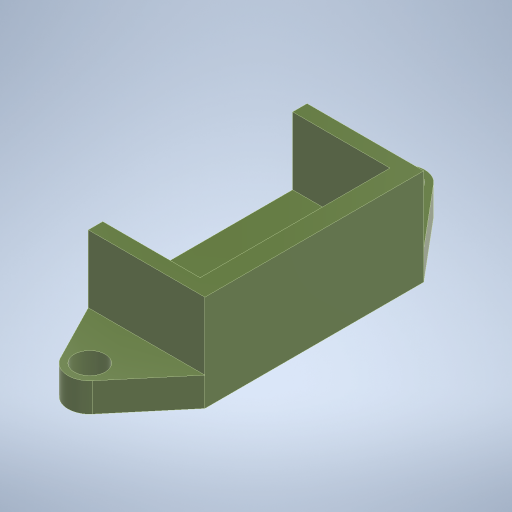
# Autodesk Inventor part: креп_концевика
Saved by Autodesk Inventor 2023.1 (Build 271208000, 208)
## iProperties
Created: 2026-01-30
Part Number: креп_концевика
Material: Типовые
Document SubType Name: Modeling
Designer: DELL
Density: 1 g/cm^3
Appearance: Темно-оливковый
Author: DELL
Autodesk Inventor part; units mm, degrees
ref_plane "YZ Plane" through (0, 0, 0) normal (1, 0, 0) x (0, 1, 0)
ref_plane "XZ Plane" through (0, 0, 0) normal (0, 1, 0) x (-1, 0, 0)
ref_plane "XY Plane" through (0, 0, 0) normal (0, 0, 1) x (1, 0, 0)
sketch "Эскиз1" plane through (0, 0, 0) normal (0, 1, 0) x (-1, 0, 0)
  line L0 (5.05, 9.85) -> (-5.05, 9.85)
  line L1 (-5.05, 9.85) -> (-5.05, -9.85)
  line L2 (-5.05, -9.85) -> (5.05, -9.85)
  line L3 (5.05, -9.85) -> (5.05, 9.85)
  line L4 (5.05, 9.85) -> (-5.05, -9.85) construction
  line L5 (-5.05, 9.85) -> (5.05, -9.85) construction
  line L6 (7.05, -11.35) -> (5.05, -11.35) construction
  line L7 (-7.05, -11.35) -> (-7.05, 11.35)
  line L8 (-7.05, 11.35) -> (5.05, 11.35)
  line L9 (7.05, 11.35) -> (7.05, -11.35) construction
  line L10 (5.05, 9.85) -> (5.05, 11.35)
  line L11 (5.05, -9.85) -> (5.05, -11.35)
  line L12 (5.05, 11.35) -> (7.05, 11.35) construction
  line L13 (5.05, -11.35) -> (-7.05, -11.35)
  point P0 (0, 0)
  dimension "d0" = 10.1
  dimension "d1" = 19.7
  dimension "d2" = 1.5
  dimension "d24" = 1.5
  constraints: 28 end point, 7 parallel, 5 perpendicular, 3 point on line, 2 midpoint, 1 horizontal
  measures "d0" distance of L2.end L1.end
  measures "d1" distance of L1.end L0.end
  measures "d2" distance between parallel lines of L2 L6
  measures "d24" distance between parallel lines of L8 L0
extrude "Выдавливание1" add sketch "Эскиз1" along normal blind 10 contours L0 L1 L2 L11 L13 L7 L8 L10
sketch "Эскиз2" plane through (0, 0, 0) normal (0, -1, 0) x (1, 0, 0)
  line L0 (-5.05, 11.35) -> (7.05, 11.35) projected
  line L1 (7.05, 11.35) -> (-5.05, 11.35)
  line L2 (-5.05, 11.35) -> (-5.05, -11.35)
  line L3 (-5.05, -11.35) -> (7.05, -11.35)
  line L4 (7.05, -11.35) -> (7.05, 11.35)
  line L5 (0, 16.25) -> (0, -16.25)
  circle A0 centre (0, 16.25) radius 2.25
  circle A1 centre (0, -16.25) radius 2.25
  line L6 (1.7234, 17.6965) -> (7.05, 11.35)
  line L7 (-5.05, 11.35) -> (-2.0009, 17.279)
  line L8 (7.05, -11.35) -> (-5.05, -11.35) projected
  line L9 (7.05, -11.35) -> (1.7234, -17.6965)
  line L10 (-5.05, -11.35) -> (-2.0009, -17.279)
  circle A2 centre (0, 16.25) radius 1.6
  circle A3 centre (0, -16.25) radius 1.6
  circle A4 centre (2.55, -4.75) radius 1.3
  circle A5 centre (2.55, 4.75) radius 1.3
  line L11 (5.05, -9.85) -> (5.05, 9.85) projected
  line L12 (2.55, -4.75) -> (2.55, 4.75)
  line L13 (0, 0) -> (7.05, 0)
  line L14 (7.05, 11.35) -> (7.05, -11.35) projected
  point P0 (-5.05, 11.35)
  point P1 (2.55, 0)
  point P2 (-5.05, 11.35)
  dimension "d5" = 32.5
  dimension "d6" = 4.5
  dimension "d10" = 4.5
  dimension "d12" = 3.2
  dimension "d13" = 3.2
  dimension "d16" = 2.6
  dimension "d17" = 2.6
  dimension "d18" = 2.5
  dimension "d19" = 2.5
  dimension "d20" = 9.5
  constraints: 22 end point, 6 centre point, 4 point on circle, 4 tangent, 3 coincident, 3 midpoint, 2 parallel, 1 horizontal, 1 perpendicular, 1 point on line, 1 vertical
  measures "d5" distance of L5.start L5.end
  measures "d6" diameter of A0
  measures "d10" diameter of A1
  measures "d12" diameter of A2
  measures "d13" diameter of A3
  measures "d16" diameter of A4
  measures "d17" diameter of A5
  measures "d18" distance from line of L11 L12.start
  measures "d19" distance from line of L11 L12.end
  measures "d20" distance of L12.start L12.end
extrude "Выдавливание2" add sketch "Эскиз2" against normal blind 3
chamfer "Фаска1" distance 1.5 angle 45 2 edges at (1.25, 0, -4.75) (1.25, 0, 4.75)
